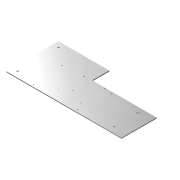
# Autodesk Inventor part: SupportsheetEPS
Saved by Autodesk Inventor 2017 (Build 210142000, 142)
## iProperties
Created: 2016-11-08
Part Number: SupportsheetEPS
Material: Aluminum 6061
Document SubType Name: Modeling
Designer: Jonis
Density: 2.7 g/cm^3
Appearance: Aluminum - Flat
Author: Jonis
Autodesk Inventor part; units mm, degrees
ref_plane "YZ Plane" through (0, 0, 0) normal (1, 0, 0) x (0, 1, 0)
ref_plane "XZ Plane" through (0, 0, 0) normal (0, 1, 0) x (-1, 0, 0)
ref_plane "XY Plane" through (0, 0, 0) normal (0, 0, 1) x (1, 0, 0)
sketch "Sketch1" plane through (0, 0, 0) normal (0, 0, 1) x (1, 0, 0)
  line L0 (0, 0) -> (380, 0)
  line L1 (380, 0) -> (380, 124)
  line L2 (380, 124) -> (179, 124)
  line L3 (179, 124) -> (179, 184)
  line L4 (179, 184) -> (0, 184)
  line L5 (0, 184) -> (0, 0)
  dimension "d0" = 380
  dimension "d1" = 124
  dimension "d2" = 201
  dimension "d3" = 60
  constraints: 12 end point, 3 perpendicular, 2 vertical, 1 horizontal
  measures "d0" distance of L0.start L0.end
  measures "d1" distance of L0.end L1.end
  measures "d2" distance of L1.end L2.end
  measures "d3" distance of L2.end L3.end
extrude "Extrusion1" add sketch "Sketch1" along normal blind 3
sketch "Sketch2" plane through (0, 0, 3) normal (0, 0, 1) x (1, 0, 0)
  line L0 (0, 184) -> (0, 0) projected
  line L1 (179, 184) -> (0, 184) projected
  line L2 (0, 0) -> (380, 0) projected
  line L3 (380, 0) -> (380, 124) projected
  line L4 (380, 124) -> (179, 124) projected
  point P0 (20, 20)
  point P1 (20, 164)
  point P2 (360, 104)
  point P3 (360, 20)
  dimension "d6" = 20
  dimension "d7" = 20
  dimension "d8" = 20
  dimension "d9" = 20
  dimension "d10" = 20
  dimension "d11" = 20
  dimension "d12" = 20
  dimension "d13" = 20
  measures "d6" distance from line of L0 point (20, 20)
  measures "d7" distance from line of L0 point (20, 164)
  measures "d8" distance from line of point (20, 164) L1
  measures "d9" distance from line of L2 point (20, 20)
  measures "d10" distance from line of L3 point (360, 20)
  measures "d11" distance from line of L2 point (360, 20)
  measures "d12" distance from line of L3 point (360, 104)
  measures "d13" distance from line of L4 point (360, 104)
hole "Hole1" at (20, 20, 3) at (20, 164, 3) at (360, 104, 3) at (360, 20, 3) direction (0, 0, -1) diameter 7 end through all
sketch "Sketch3" plane through (0, 0, 3) normal (0, 0, 1) x (1, 0, 0)
  line L0 (0, 0) -> (380, 0) projected
  line L1 (0, 184) -> (0, 0) projected
  point P0 (153.17, 121.31)
  point P1 (226.83, 121.31)
  dimension "d21" = 73.66
  dimension "d22" = 121.31
  dimension "d23" = 121.31
  dimension "d24" = 153.17
  measures "d21" distance of point (226.83, 121.31) point (153.17, 121.31)
  measures "d22" distance from line of L0 point (153.17, 121.31)
  measures "d23" distance from line of L0 point (226.83, 121.31)
  measures "d24" distance from line of L1 point (153.17, 121.31)
hole "Hole2" at (153.17, 121.31, 3) at (226.83, 121.31, 3) direction (0, 0, -1) diameter 3.5 end through all
sketch "Sketch4" plane through (380, 0, 0) normal (1, 0, 0) x (0, 0, -1)
  line L0 (0, 124) -> (-3, 124) projected
  line L1 (0, 0) -> (-3, 0)
  line L2 (-3, 0) -> (-3, 124)
  line L3 (-3, 124) -> (0, 124)
  line L4 (0, 124) -> (0, 0)
  constraints: 8 end point, 2 parallel, 1 horizontal, 1 perpendicular
extrude "Extrusion2" add sketch "Sketch4" along normal blind 26
sketch "Sketch5" plane through (0, 0, 3) normal (0, 0, 1) x (1, 0, 0)
  circle A0 centre (241.7805, 9.3195) radius 2.5 projected
  circle A1 centre (175.7805, 60.3195) radius 2.5 projected
  circle A2 centre (254.2805, 116.8195) radius 2.5 projected
  circle A3 centre (79.2805, 116.8195) radius 2.5 projected
  circle A4 centre (89.2805, 6.8195) radius 2.5 projected
  line L0 (179, 124) -> (406, 124) projected
  line L1 (179, 184) -> (0, 184) projected
  line L2 (0, 184) -> (0, 0) projected
  dimension "d65" = 7.1805
  dimension "d66" = 7.1805
  dimension "d67" = 67.1805
  dimension "d68" = 114.6805
  dimension "d69" = 63.6805
  dimension "d70" = 117.1805
  dimension "d71" = 177.1805
  dimension "d72" = 79.2805
  dimension "d73" = 89.2805
  dimension "d74" = 175.7805
  dimension "d75" = 241.7805
  dimension "d76" = 254.2805
  constraints: 5 coincident
  measures "d65" distance from line of point (254.28, 116.819) L0
  measures "d66" distance from line of L0 point (79.28, 116.819)
  measures "d67" distance from line of L1 point (79.28, 116.819)
  measures "d68" distance from line of L0 point (241.78, 9.319)
  measures "d69" distance from line of L0 point (175.78, 60.32)
  measures "d70" distance from line of L0 point (89.281, 6.82)
  measures "d71" distance from line of point (89.281, 6.82) L1
  measures "d72" distance from line of A3.centre L2
  measures "d73" distance from line of L2 point (89.281, 6.82)
  measures "d74" distance from line of L2 point (175.78, 60.32)
  measures "d75" distance from line of L2 point (241.78, 9.319)
  measures "d76" distance from line of L2 point (254.28, 116.819)
hole "Hole3" at (241.7805, 9.3195, 3) at (254.2805, 116.8195, 3) at (175.7805, 60.3195, 3) at (89.2805, 6.8195, 3) at (79.2805, 116.8195, 3) direction (0, 0, -1) diameter 3.242 depth 5 tip angle 118 thread size "M4x0.7" class "6H" standard "ISO Metric profile"
sketch "Sketch6" plane through (0, 0, 3) normal (0, 0, 1) x (1, 0, 0)
  circle A0 centre (225.65, 120.31) radius 1.75 projected
  circle A1 centre (151.99, 120.31) radius 1.75 projected
  point P0 (0, 0)
  constraints: 2 coincident
hole "Hole4" at (225.65, 120.31, 3) at (151.99, 120.31, 3) direction (0, 0, -1) diameter 3 depth 5 tip angle 118
sketch "Sketch7" plane through (0, 0, 3) normal (0, 0, 1) x (1, 0, 0)
  circle A0 centre (151.99, 120.31) radius 1.75 projected
  circle A1 centre (225.65, 120.31) radius 1.75 projected
  line L0 (179, 124) -> (406, 124) projected
  line L1 (0, 184) -> (0, 0) projected
  point P0 (228.19, 34.585)
  point P1 (148.18, 34.585)
  dimension "d48" = 85.725
  dimension "d49" = 85.725
  dimension "d50" = 80.01
  dimension "d51" = 2.54
  dimension "d52" = 3.69
  dimension "d53" = 89.415
  dimension "d54" = 151.99
  dimension "d55" = 148.18
  dimension "d56" = 73.66
  dimension "d57" = 228.19
  measures "d48" vertical distance of A1.centre point (228.19, 34.585)
  measures "d49" vertical distance of A0.centre point (148.18, 34.585)
  measures "d50" distance of point (148.18, 34.585) point (228.19, 34.585)
  measures "d51" horizontal distance of point (228.19, 34.585) A1.centre
  measures "d52" distance from line of A1.centre L0
  measures "d53" distance from line of L0 point (148.18, 34.585)
  measures "d54" distance from line of L1 A0.centre
  measures "d55" distance from line of L1 point (148.18, 34.585)
  measures "d56" distance of A0.centre A1.centre
  measures "d57" distance from line of L1 point (228.19, 34.585)
hole "Hole5" at (228.19, 34.585, 3) at (148.18, 34.585, 3) direction (0, 0, -1) diameter 2.5 depth 5 tip angle 118
body "Solid1"
